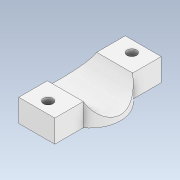
# Autodesk Inventor part: soporte_flauta_4
Saved by Autodesk Inventor 2022 (Build 260153000, 153)
## iProperties
Created: 2022-05-10
Part Number: soporte_flauta_4
Material: Generic
Document SubType Name: Modeling
Designer: ferna
Density: 1 g/cm^3
Appearance: Snow
Author: ferna
Autodesk Inventor part; units mm, degrees
ref_plane "YZ Plane" through (0, 0, 0) normal (1, 0, 0) x (0, 1, 0)
sketch "Sketch1" plane through (0, 0, 0) normal (0, 1, 0) x (-1, 0, 0)
  circle A0 centre (0, 0) radius 14
  circle A1 centre (0, 0) radius 11
  dimension "d0" = 28
  dimension "d1" = 22
  constraints: 2 centre point, 2 coincident
  measures "d0" diameter of A0
  measures "d1" diameter of A1
extrude "Extrusion1" add sketch "Sketch1" along normal blind 10
sketch "Sketch2" plane through (0, 10, 0) normal (0, 1, 0) x (1, 0, 0)
  circle A0 centre (0, 0) radius 17.5
  dimension "d4" = 35
  constraints: 1 centre point, 1 coincident
  measures "d4" diameter of A0
extrude "Extrusion2" add sketch "Sketch2" along normal blind 3
sketch "Sketch3" plane through (0, 0, 0) normal (1, 0, 0) x (0, 1, 0)
  line L0 (13, -17.5) -> (13, 17.5) projected
  line L1 (13, 0) -> (28, 0)
  circle A0 centre (28, 0) radius 15
  line L2 (28, -15) -> (28, -17.5)
  line L3 (28, -17.5) -> (13, -17.5)
  line L4 (13, -17.5) -> (13, 17.5)
  line L5 (13, 17.5) -> (28, 17.5)
  line L6 (10, 17.5) -> (13, 17.5) projected
  line L7 (28, 17.5) -> (28, 15)
  point P0 (0, 0)
  dimension "d7" = 15
  constraints: 12 end point, 3 point on circle, 2 collinear, 2 point on line, 1 centre point, 1 coincident, 1 horizontal, 1 midpoint, 1 perpendicular, 1 vertical
  measures "d7" distance of L1.start L1.end
extrude "Extrusion3" add sketch "Sketch3" along normal up to surface contours L0 A0 L2 L3 | L0 L5 L7 A0 round surface about axis through (0, 10, 0) along (0, 1, 0) radius 17.5 far side no
sketch "Sketch4" plane through (0, 0, 0) normal (-1, 0, 0) x (0, 0, 1)
  line L0 (-17.5, 28) -> (-15, 28) projected
  line L1 (-17.5, 13) -> (-17.5, 28) projected
  line L2 (0, 13) -> (-17.5, 13) projected
  arc A0 (-15, 28) -> (0, 13) centre (0, 28) ccw projected
  line L3 (17.5, 13) -> (0, 13) projected
  line L4 (17.5, 13) -> (17.5, 28) projected
  line L5 (15, 28) -> (17.5, 28) projected
  arc A1 (0, 13) -> (15, 28) centre (0, 28) ccw projected
  point P0 (0, 0)
extrude "Extrusion4" add sketch "Sketch4" along normal up to surface round surface about axis through (0, 10, 0) along (0, 1, 0) radius 17.5 far side no
sketch "Sketch5" plane through (0, 0, 0) normal (0, 0, 1) x (1, 0, 0)
  line L0 (-9.0139, 28) -> (9.0139, 28) projected
  line L1 (0, 28) -> (0, 25)
  line L2 (0, 25) -> (5, 25)
  line L3 (5, 25) -> (5, 23)
  line L4 (5, 23) -> (-5, 23)
  line L5 (-5, 23) -> (-5, 25)
  line L6 (-5, 25) -> (0, 25)
  point P0 (0, 0)
  dimension "d12" = 3
  dimension "d13" = 5
  dimension "d14" = 2
  dimension "d15" = 10
  constraints: 12 end point, 5 perpendicular, 1 midpoint, 1 point on line, 1 vertical
  measures "d12" distance of L1.start L1.end
  measures "d13" distance of L1.end L2.end
  measures "d14" distance of L2.end L3.end
  measures "d15" distance of L3.end L4.end
extrude "Extrusion5" cut sketch "Sketch5" along normal through all both and the other way through all
sketch "Sketch6" plane through (0, 10, 0) normal (0, -1, 0) x (1, 0, 0)
  circle A0 centre (0, 0) radius 14 projected
  circle A1 centre (0, 0) radius 14.5
  dimension "d18" = 29
  constraints: 1 centre point, 1 coincident
  measures "d18" diameter of A1
extrude "Extrusion6" add sketch "Sketch6" along normal up to surface (10 mm away)
ref_plane "Work Plane1" through (0, 25, 17.5) normal (0, 0, 1) x (1, 0, 0)
sketch "Sketch7" plane through (0, 25, 17.5) normal (0, 0, 1) x (1, 0, 0)
  line L0 (5, -2) -> (-5, -2) projected
  line L1 (5, -2) -> (13.7117, -2)
  line L2 (13.7117, -2) -> (0, 13.5732)
  line L3 (0, 13.5732) -> (-17.6873, -2)
  line L4 (-17.6873, -2) -> (5, -2)
  point P0 (0, -25)
  constraints: 8 end point, 1 collinear, 1 horizontal, 1 perpendicular, 1 point on line
extrude "Extrusion7" cut sketch "Sketch7" against normal through all
sketch "Sketch8" plane through (0, 25, 17.5) normal (0, 0, 1) x (1, 0, 0)
  line L0 (-10.3078, -2) -> (10.3078, -2) projected
  line L1 (-10.3078, -2) -> (10.3078, -2) projected
  line L2 (17.5, -12) -> (-17.5, -12) projected
  line L3 (-10.3078, -2) -> (10.3078, -2)
  line L4 (10.3078, -2) -> (10.3078, -12)
  line L5 (10.3078, -12) -> (-10.3078, -12)
  line L6 (-10.3078, -12) -> (-10.3078, -2)
  point P0 (0, -25)
  constraints: 8 end point, 2 parallel, 1 horizontal, 1 perpendicular, 1 point on line
extrude "Extrusion8" add sketch "Sketch8" along normal up to surface round surface about axis through (0, 10, 0) along (0, 1, 0) radius 17.5 far side no
sketch "Sketch9" plane through (0, 25, 17.5) normal (0, 0, 1) x (1, 0, 0)
  line L0 (10.3078, -2) -> (-10.3078, -2) projected
  line L1 (-10.3078, -2) -> (-10.3078, -12) projected
  line L2 (-10.3078, -12) -> (0, -12) projected
  line L3 (0, -12) -> (10.3078, -12) projected
  line L4 (10.3078, -12) -> (10.3078, -2) projected
  point P0 (0, -25)
extrude "Extrusion9" add sketch "Sketch9" along normal blind 13
sketch "Sketch10" plane through (0, 13, 0) normal (0, -1, 0) x (1, 0, 0)
  line L0 (2.4537, 28.25) -> (4.9075, 24)
  line L1 (-2.4537, 28.25) -> (2.4537, 28.25)
  line L2 (-4.9075, 24) -> (-2.4537, 28.25)
  line L3 (-2.4537, 19.75) -> (-4.9075, 24)
  line L4 (2.4537, 19.75) -> (-2.4537, 19.75)
  line L5 (4.9075, 24) -> (2.4537, 19.75)
  circle A0 centre (0, 24) radius 2.75
  circle A1 centre (0, 0) radius 17.5 projected
  line L6 (0, 17.5) -> (0, 30.5)
  line L7 (-10.3078, 30.5) -> (10.3078, 30.5) projected
  constraints: 14 end point, 2 midpoint, 1 centre point, 1 vertical alignment, 1 other
extrude "Extrusion10" cut sketch "Sketch10" against normal blind 3.8 contours L0 L5 L4 L6 A0 L1 | L6 A0 L4 L3 L2 L1
sketch "Sketch11" plane through (0, 13, 24) normal (0, -1, 0) x (1, 0, 0)
  circle A0 centre (0, 0) radius 2.75 projected
  point P0 (0, -24)
extrude "Extrusion11" cut sketch "Sketch11" against normal through all
ref_plane "Work Plane2" through (0, 10, -17.5) normal (0, 0, 1) x (1, 0, 0)
sketch "Sketch12" plane through (0, 10, -17.5) normal (0, 0, 1) x (1, 0, 0)
  line L0 (-10.3078, 13) -> (-10.3078, 3) projected
  line L1 (-10.3078, 3) -> (10.3078, 3) projected
  line L2 (10.3078, 3) -> (10.3078, 13) projected
  line L3 (10.3078, 13) -> (-10.3078, 13) projected
  point P0 (0, -10)
extrude "Extrusion12" add sketch "Sketch12" along normal up to surface round surface about axis through (0, 10, 0) along (0, 1, 0) radius 17.5 far side no
sketch "Sketch13" plane through (0, 10, -17.5) normal (0, 0, -1) x (-1, 0, 0)
  line L0 (-10.3078, 13) -> (10.3078, 13) projected
  line L1 (-10.3078, 3) -> (-10.3078, 13) projected
  line L2 (0, 3) -> (-10.3078, 3) projected
  line L3 (10.3078, 3) -> (0, 3) projected
  line L4 (10.3078, 13) -> (10.3078, 3) projected
  point P0 (0, -10)
extrude "Extrusion13" add sketch "Sketch13" along normal blind 13
sketch "Sketch14" plane through (0, 13, 0) normal (0, -1, 0) x (1, 0, 0)
  circle A0 centre (0, 0) radius 17.5 projected
  line L0 (0, -17.5) -> (0, -30.5)
  line L1 (-10.3078, -30.5) -> (10.3078, -30.5) projected
  line L2 (-4.9075, 24) -> (-2.4537, 28.25) projected
  line L3 (-2.4537, 19.75) -> (-4.9075, 24) projected
  line L4 (2.4537, 19.75) -> (-2.4537, 19.75) projected
  line L5 (4.9075, 24) -> (2.4537, 19.75) projected
  line L6 (2.4537, 28.25) -> (4.9075, 24) projected
  line L7 (-2.4537, 28.25) -> (2.4537, 28.25) projected
  circle A1 centre (0, 24) radius 2.75 projected
  line L8 (-4.9075, -24) -> (-2.4537, -19.75)
  line L9 (-2.4537, -28.25) -> (-4.9075, -24)
  line L10 (2.4537, -28.25) -> (-2.4537, -28.25)
  line L11 (4.9075, -24) -> (2.4537, -28.25)
  line L12 (2.4537, -19.75) -> (4.9075, -24)
  line L13 (-2.4537, -19.75) -> (2.4537, -19.75)
  circle A2 centre (0, -24) radius 2.75
  constraints: 14 end point, 2 midpoint, 1 centre point, 1 vertical alignment, 1 other
extrude "Extrusion14" cut sketch "Sketch14" against normal blind 3.8 contours L13 L12 L11 L10 L0 A2 | L0 A2 L10 L9 L8 L13
sketch "Sketch15" plane through (0, 13, 0) normal (0, -1, 0) x (1, 0, 0)
  circle A0 centre (0, -24) radius 2.75 projected
  point P0 (0, 0)
extrude "Extrusion15" cut sketch "Sketch15" against normal through all
sketch "Sketch16" plane through (0, 0, 0) normal (0, -1, 0) x (1, 0, 0)
  circle A0 centre (0, 0) radius 14.5 projected
  circle A1 centre (0, 0) radius 11 projected
extrude "Extrusion16" cut sketch "Sketch16" against normal up to surface (10 mm away)
sketch "Sketch17" plane through (0, 16.8, 0) normal (0, -1, 0) x (1, 0, 0)
  line L0 (-4.9075, 24) -> (-2.4537, 28.25) projected
  line L1 (-2.4537, 19.75) -> (-4.9075, 24) projected
  line L2 (2.4537, 19.75) -> (-2.4537, 19.75) projected
  line L3 (4.9075, 24) -> (2.4537, 19.75) projected
  line L4 (2.4537, 28.25) -> (4.9075, 24) projected
  line L5 (-2.4537, 28.25) -> (2.4537, 28.25) projected
  circle A0 centre (0, 24) radius 2.75 projected
  line L6 (4.9075, -24) -> (2.4537, -28.25) projected
  line L7 (2.4537, -19.75) -> (4.9075, -24) projected
  line L8 (-2.4537, -19.75) -> (2.4537, -19.75) projected
  line L9 (-4.9075, -24) -> (-2.4537, -19.75) projected
  line L10 (-2.4537, -28.25) -> (-4.9075, -24) projected
  line L11 (2.4537, -28.25) -> (-2.4537, -28.25) projected
  circle A1 centre (0, -24) radius 2.75 projected
  point P0 (0, 0)
extrude "Extrusion17" add sketch "Sketch17" along normal up to surface (3.8 mm away)
sketch "Sketch18" plane through (0, 13, 0) normal (0, -1, 0) x (1, 0, 0)
  circle A0 centre (0, 24) radius 2.75 projected
  circle A1 centre (0, -24) radius 2.75 projected
  circle A2 centre (0, 24) radius 4.25
  circle A3 centre (0, -24) radius 4.25
  point P0 (0, 0)
  dimension "d43" = 8.5
  dimension "d44" = 8.5
  constraints: 2 centre point, 2 coincident
  measures "d43" diameter of A2
  measures "d44" diameter of A3
extrude "Extrusion18" cut sketch "Sketch18" against normal blind 2.7
sketch "Sketch19" plane through (0, 13, 0) normal (0, -1, 0) x (1, 0, 0)
  circle A0 centre (0, -24) radius 4.25 projected
  arc A1 (-10.3078, -14.1421) -> (10.3078, -14.1421) centre (0, 0) ccw projected
  line L0 (-10.3078, -14.1421) -> (-10.3078, -30.5) projected
  line L1 (10.3078, -30.5) -> (-10.3078, -30.5) projected
  line L2 (10.3078, -30.5) -> (10.3078, -14.1421) projected
  circle A2 centre (0, 24) radius 4.25 projected
  arc A3 (10.3078, 14.1421) -> (-10.3078, 14.1421) centre (0, 0) ccw projected
  line L3 (10.3078, 14.1421) -> (10.3078, 30.5) projected
  line L4 (-10.3078, 30.5) -> (10.3078, 30.5) projected
  line L5 (-10.3078, 30.5) -> (-10.3078, 14.1421) projected
extrude "Extrusion19" add sketch "Sketch19" along normal up to surface (3 mm away)
sketch "Sketch20" plane through (0, 15.7, -24) normal (0, -1, 0) x (1, 0, 0)
  circle A0 centre (0, 0) radius 4.25 projected
  circle A1 centre (0, 0) radius 2.75 projected
  circle A2 centre (0, 48) radius 4.25 projected
  circle A3 centre (0, 48) radius 2.75 projected
  point P0 (0, 24)
extrude "Extrusion20" add sketch "Sketch20" along normal blind 3
body "Solid1"
